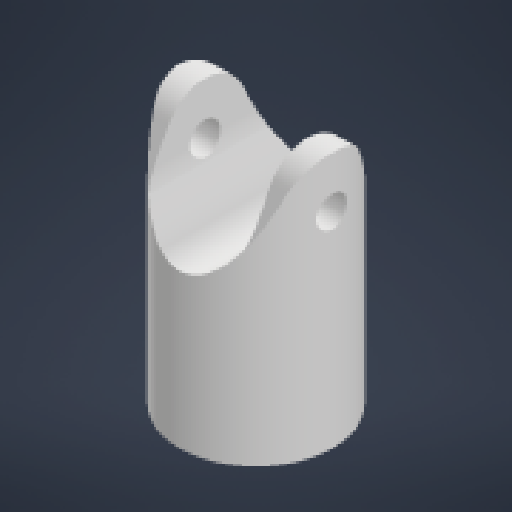
# Autodesk Inventor part: Base_joint
Saved by Autodesk Inventor 2026.2 (Build 302298010, 298A)
## iProperties
Created: 2026-06-25
Part Number: Base_joint
Material: Generic
Document SubType Name: Modeling
Designer: frede
Density: 1 g/cm^3
Appearance: Default
Author: frede
Autodesk Inventor part; units mm, degrees
ref_plane "YZ Plane" through (0, 0, 0) normal (1, 0, 0) x (0, 1, 0)
ref_plane "XZ Plane" through (0, 0, 0) normal (0, 1, 0) x (-1, 0, 0)
ref_plane "XY Plane" through (0, 0, 0) normal (0, 0, 1) x (1, 0, 0)
sketch "Sketch1" plane through (0, 0, 0) normal (0, 1, 0) x (-1, 0, 0)
  circle A0 centre (0, 0) radius 4.925
  arc A1 (3.9454, 1.0194) -> (-3.5041, 2.0801) centre (0, 0) ccw
  line L0 (2.6068, 1.21) -> (3.9454, 1.0194)
  line L1 (2.1655, -1.8895) -> (2.6068, 1.21)
  line L2 (3.5041, -2.0801) -> (2.1655, -1.8895)
  arc A2 (-3.9454, -1.0194) -> (3.5041, -2.0801) centre (0, 0) ccw
  line L3 (-2.6068, -1.21) -> (-3.9454, -1.0194)
  line L4 (-2.1655, 1.8895) -> (-2.6068, -1.21)
  line L5 (-3.5041, 2.0801) -> (-2.1655, 1.8895)
  circle A3 centre (0, 0.038) radius 7.5
  dimension "d4" = 15
  constraints: 12 end point, 4 centre point, 4 point on circle
  measures "d4" diameter of A3
extrude "Extrusion1" add sketch "Sketch1" along normal blind 15 contours A0 | A3
sketch "Sketch2" plane through (0, 15, 0) normal (0, 1, 0) x (1, 0, 0)
  line L0 (-3.9454, -1.0194) -> (-2.6068, -1.21) projected
  line L1 (-2.6068, -1.21) -> (-2.1655, 1.8895) projected
  line L2 (-2.1655, 1.8895) -> (-3.5041, 2.0801) projected
  arc A0 (3.9454, 1.0194) -> (-3.5041, 2.0801) centre (0, 0) ccw projected
  line L3 (3.9454, 1.0194) -> (2.6068, 1.21) projected
  line L4 (2.6068, 1.21) -> (2.1655, -1.8895) projected
  line L5 (2.1655, -1.8895) -> (3.5041, -2.0801) projected
  arc A1 (-3.9454, -1.0194) -> (3.5041, -2.0801) centre (0, 0) ccw projected
  circle A2 centre (0, -0.038) radius 7.5 projected
extrude "Extrusion2" add sketch "Sketch2" along normal blind 10 contours L0 L1 L2 A0 L3 L4 L5 A1 | A2
sketch "Sketch3" plane through (0, 0, 0) normal (1, 0, 0) x (0, 1, 0)
  line L0 (25, -7.462) -> (25, 7.538) projected
  line L1 (0, -7.462) -> (0, 7.538) projected
  line L2 (0, 7.538) -> (25, 7.538) projected
  line L3 (0, -7.462) -> (25, -7.462) projected
  line L4 (25, 0.038) -> (17, 0.038)
  circle A0 centre (21, 0.038) radius 4
  line L5 (25, 7.538) -> (15, 7.538)
  line L6 (15, 7.538) -> (22.7991, 3.6106)
  line L7 (25, -7.462) -> (15, -7.462)
  line L8 (15, -7.462) -> (22.7991, -3.5346)
  point P0 (0, 0)
  dimension "d5" = 8
  dimension "d6" = 10
  dimension "d7" = 10
  constraints: 10 end point, 3 point on circle, 2 midpoint, 2 point on line, 2 tangent, 1 centre point, 1 horizontal
  measures "d5" distance of L4.start L4.end
  measures "d6" distance of L2.end L5.end
  measures "d7" distance of L3.end L7.end
extrude "Extrusion3" cut sketch "Sketch3" along normal mid plane 20 contours L3 L8 A0 L0 | A0 L6 L2 L0
sketch "Sketch4" plane through (0, 0, 0) normal (0, 0, 1) x (1, 0, 0)
  line L0 (6.5944, 22.7991) -> (-6.5944, 22.7991) projected
  line L1 (-6.5944, 22.7991) -> (6.5944, 22.7991) projected
  ellipse E0 centre (0, 29.8935) end of major axis (0, 15) minor radius 7.5 (-6.5944, 22.7991) -> (6.5944, 22.7991) ccw projected
  line L2 (6.5944, 22.7991) -> (-6.5944, 22.7991) projected
  line L3 (7.5, 25) -> (-7.5, 25) projected
  line L4 (-7.5, 0) -> (-7.5, 25) projected
  line L5 (7.5, 0) -> (7.5, 25) projected
  line L6 (0, 25) -> (5, 25)
  line L7 (0, 25) -> (0, 20)
  circle A0 centre (0, 20) radius 5
  line L8 (-5, 25) -> (-5, 20)
  line L9 (5, 20) -> (5, 25)
  point P0 (0, 0)
  point P1 (-4.6939, 18.2775)
  point P2 (4.6939, 18.2775)
  dimension "d10" = 5
  dimension "d11" = 5
  constraints: 8 end point, 3 point on circle, 2 point on line, 2 tangent, 1 centre point, 1 coincident, 1 midpoint, 1 parallel, 1 vertical, 6 other
  measures "d10" distance of L6.start L6.end
  measures "d11" distance of L6.start L7.end
extrude "Extrusion4" cut sketch "Sketch4" along normal mid plane 20 contours L9 A0 L0 | L0 A0 L3 L9 | E0 A0 L0 | L0 L7 A0 | L0 A0 L7 | A0 L0 L8 L3 | A0 L8 L0
sketch "Sketch5" plane through (0, 0, 0) normal (1, 0, 0) x (0, 1, 0)
  line L0 (25, 0.038) -> (20, 0.038)
  line L1 (20, -4.9441) -> (20, 5.0202) projected
  circle A0 centre (20, 0.038) radius 1.5
  point P0 (0, 0)
  dimension "d16" = 3
  constraints: 2 end point, 1 centre point, 1 midpoint, 2 other
  measures "d16" diameter of A0
extrude "Extrusion5" cut sketch "Sketch5" along normal mid plane 20
sketch "Sketch6" plane through (0, 0, 0) normal (1, 0, 0) x (0, 1, 0)
  line L0 (17.4802, 2.5181) -> (17.52, -2.4818) projected
  line L1 (17.52, -2.4818) -> (22.5198, -2.442) projected
  line L2 (22.5198, -2.442) -> (22.48, 2.5578) projected
  line L3 (22.48, 2.5578) -> (17.4802, 2.5181) projected
  spline S0 degree 7 poles (25, 0.038) (25, 0.1961) (24.9927, 0.3539) (24.9782, 0.5106) (24.9566, 0.6656) (24.9282, 0.8178) (24.8936, 0.9667) (24.8294, 1.1973) (24.8034, 1.2817) (24.7756, 1.3647) (24.7459, 1.4462) (24.7145, 1.5262) (24.6815, 1.6046) (24.4666, 2.0813) (24.2449, 2.4366) (23.9933, 2.7484) (23.7191, 3.0193) (23.4273, 3.252) (23.1203, 3.4489) (22.7991, 3.6106) knots 0 0 0 0 0 0 0 0 0.213658 0.213658 0.213658 0.213658 0.213658 0.213658 0.340268 0.340268 0.340268 0.340268 0.340268 0.340268 1 1 1 1 1 1 1 1 projected
  line L4 (22.7991, 3.6106) -> (18.2775, 5.8876) projected
  line L5 (18.2775, 5.8876) -> (18.2775, 5.8876) projected
  line L6 (18.2775, 5.8876) -> (22.7991, 3.6106) projected
  spline S1 degree 7 poles (25, 0.038) (25, -0.12) (24.9927, -0.2778) (24.9782, -0.4346) (24.9566, -0.5895) (24.9282, -0.7418) (24.8936, -0.8907) (24.8294, -1.1212) (24.8034, -1.2057) (24.7756, -1.2886) (24.7459, -1.3701) (24.7145, -1.4501) (24.6815, -1.5285) (24.4666, -2.0052) (24.2449, -2.3606) (23.9933, -2.6723) (23.7191, -2.9432) (23.4273, -3.176) (23.1203, -3.3728) (22.7991, -3.5346) knots 0 0 0 0 0 0 0 0 0.213658 0.213658 0.213658 0.213658 0.213658 0.213658 0.340268 0.340268 0.340268 0.340268 0.340268 0.340268 1 1 1 1 1 1 1 1 projected
  line L7 (22.7991, -3.5346) -> (18.2775, -5.8115) projected
  line L8 (18.2775, -5.8115) -> (18.2775, -5.8115) projected
  line L9 (18.2775, -5.8115) -> (22.7991, -3.5346) projected
  line L10 (0, -7.462) -> (0, 7.538) projected
  line L11 (22.7991, 3.6106) -> (14.7991, 3.6106)
  line L12 (22.7991, 3.6106) -> (30.7991, 3.6106) construction
  line L13 (22.7991, -3.5346) -> (14.7991, -3.5346)
  line L14 (22.7991, -3.5346) -> (30.7991, -3.5346) construction
  line L15 (14.7991, -3.5346) -> (14.7991, 3.6106)
  line L16 (22.48, 2.5578) -> (22.63, 2.5578)
  line L17 (22.63, 2.5578) -> (22.63, 2.7078)
  line L18 (22.63, 2.7078) -> (22.48, 2.7078)
  line L19 (22.48, 2.7078) -> (22.48, 2.5578)
  line L20 (17.52, -2.4818) -> (17.37, -2.4818)
  line L21 (17.37, -2.4818) -> (17.37, -2.6318)
  line L22 (17.37, -2.6318) -> (17.52, -2.6318)
  line L23 (17.52, -2.6318) -> (17.52, -2.4818)
  line L24 (17.37, -2.6318) -> (22.63, -2.6318)
  line L25 (22.63, -2.6318) -> (22.63, 2.7078)
  line L26 (22.63, 2.7078) -> (17.37, 2.7078)
  line L27 (17.37, 2.7078) -> (17.37, -2.6318)
  point P0 (0, 0)
  point P1 (22.7991, 3.6106)
  point P2 (22.7991, -3.5346)
  point P3 (25, 0.038)
  dimension "d17" = 8
  dimension "d18" = 180
  dimension "d19" = 8
  dimension "d20" = 180
  dimension "d21" = 0.15
  dimension "d22" = 0.15
  dimension "d23" = 0.15
  dimension "d24" = 0.15
  constraints: 34 end point, 7 horizontal, 6 parallel, 3 perpendicular, 2 collinear, 6 other
  measures "d17" distance of L6.end L11.end
  measures "d18" angle of L11 L12
  measures "d19" distance of L9.end L13.end
  measures "d20" angle of L13 L14
  measures "d21" distance of L18.end L17.end
  measures "d22" distance of L17.end L16.end
  measures "d23" distance of L22.end L21.end
  measures "d24" distance of L21.end L20.end
extrude "Extrusion6" add sketch "Sketch6" along normal mid plane 20
sketch "Sketch7" plane through (0, 0, 0) normal (0, 0, 1) x (1, 0, 0)
  line L0 (6.5944, 14.7991) -> (6.5944, 22.7991) projected
  ellipse E0 centre (0, 29.8935) end of major axis (0, 15) minor radius 7.5 (4.6939, 18.2775) -> (6.5944, 22.7991) ccw projected
  ellipse E1 centre (0, 29.8935) end of major axis (0, 15) minor radius 7.5 (-4.6939, 18.2775) -> (4.6939, 18.2775) ccw projected
  ellipse E2 centre (0, 29.8935) end of major axis (0, 15) minor radius 7.5 (-6.5944, 22.7991) -> (-4.6939, 18.2775) ccw projected
  line L1 (-6.5944, 22.7991) -> (-6.5944, 14.7991) projected
  line L2 (-6.5944, 14.7991) -> (-6.5944, 14.7991) projected
  line L3 (-6.5944, 14.7991) -> (-6.5944, 22.7991) projected
  ellipse E3 centre (0, 29.8935) end of major axis (0, 44.787) minor radius 7.5 (-6.5944, 22.7991) -> (-4.6939, 18.2775) ccw projected
  ellipse E4 centre (0, 29.8935) end of major axis (0, 44.787) minor radius 7.5 (-4.6939, 18.2775) -> (4.6939, 18.2775) ccw projected
  ellipse E5 centre (0, 29.8935) end of major axis (0, 44.787) minor radius 7.5 (4.6939, 18.2775) -> (6.5944, 22.7991) ccw projected
  line L4 (6.5944, 22.7991) -> (6.5944, 14.7991) projected
  line L5 (6.5944, 14.7991) -> (6.5944, 14.7991) projected
  line L6 (7.5, 0) -> (-7.5, 0) projected
  arc A0 (-5, 20) -> (-4.6939, 18.2775) centre (0, 20) ccw projected
  ellipse E6 centre (0, 29.8935) end of major axis (0, 44.787) minor radius 7.5 (-6.5944, 22.7991) -> (-4.6939, 18.2775) ccw projected
  line L7 (-6.5944, 22.7991) -> (-5, 22.7991) projected
  line L8 (-5, 22.7991) -> (-5, 20) projected
  ellipse E7 centre (0, 29.8935) end of major axis (0, 44.787) minor radius 7.5 (-4.6939, 18.2775) -> (4.6939, 18.2775) ccw projected
  ellipse E8 centre (0, 29.8935) end of major axis (0, 44.787) minor radius 7.5 (4.6939, 18.2775) -> (6.5944, 22.7991) ccw projected
  line L9 (6.5944, 22.7991) -> (5, 22.7991) projected
  line L10 (6.5944, 22.7991) -> (10, 22.7991) projected
  line L11 (10, 22.7991) -> (10, 22.7991) projected
  line L12 (6.5944, 22.7991) -> (10, 22.7991) projected
  line L13 (5, 22.7991) -> (6.5944, 22.7991) projected
  line L14 (-5, 22.7991) -> (5, 22.7991) projected
  line L15 (-6.5944, 22.7991) -> (-5, 22.7991) projected
  line L16 (-10, 22.7991) -> (-6.5944, 22.7991) projected
  line L17 (-10, 22.7991) -> (-10, 22.7991) projected
  line L18 (-10, 22.7991) -> (-6.5944, 22.7991) projected
  line L19 (-5, 22.7991) -> (-6.5944, 22.7991) projected
  line L20 (-5, 22.7991) -> (5, 22.7991) projected
  line L21 (10, 25) -> (-10, 25) projected
  ellipse E9 centre (0, 29.8935) end of major axis (0, 44.787) minor radius 7.5 (-6.5944, 22.7991) -> (-4.6939, 18.2775) ccw projected
  arc A1 (4.6939, 18.2775) -> (5, 20) centre (0, 20) ccw projected
  line L22 (5, 20) -> (5, 22.7991) projected
  line L23 (-5, 22.7991) -> (-5, 20) projected
  arc A2 (-5, 20) -> (-4.6939, 18.2775) centre (0, 20) ccw projected
  line L24 (-5, 22.7991) -> (-5, 25)
  line L25 (5, 22.7991) -> (5, 25)
  point P0 (0, 0)
  point P1 (-4.6939, 18.2775)
  constraints: 4 end point, 2 perpendicular, 2 point on line, 10 other
extrude "Extrusion7" cut sketch "Sketch7" along normal mid plane 20 contours E1 A0 L8 L14 L22 A1 | L14 L24 L21 L25
body "Solid1"
